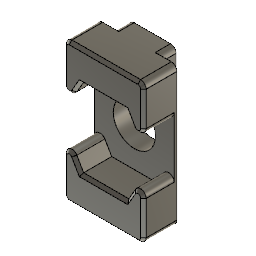
TNut_HeatExpansion v1 (Autodesk Fusion 360 design; units mm, degrees)
Autodesk Fusion 360 part; units mm, degrees
sketch "Sketch1" plane through (0, 0, 0) normal (0, 0, 1) x (1, 0, 0)
  line L0 (-2.85, 0.9) -> (-2.85, -1.5)
  line L1 (2.85, -1.5) -> (2.85, 0.9)
  line L2 (2.85, 0.9) -> (1.7, 0.9)
  line L3 (1.7, 0.9) -> (1.7, 2)
  line L4 (1.7, 2) -> (-1.7, 2)
  line L5 (-1.7, 2) -> (-1.7, 0.9)
  line L6 (-1.7, 0.9) -> (-2.85, 0.9)
  line L7 (-2.85, -1.5) -> (2.85, -1.5)
  dimension "d1" = 3.4
  dimension "d2" = 5.7
  dimension "d3" = 2.4
  dimension "d4" = 1.1
  dimension "d5" = 1.7
  dimension "d6" = 2
  dimension "d7" = 1.15
  constraint vertical L0
  constraint parallel L0 L1
  constraint perpendicular L0 L2
  constraint perpendicular L2 L3
  constraint perpendicular L3 L4
  constraint perpendicular L4 L5
  constraint perpendicular L0 L6
  constraint collinear L2 L6
  constraint perpendicular L0 L7
  measures "d1" distance of L3 L5
  measures "d2" distance of L0 L1
  measures "d3" distance of L0.start L0.end
  measures "d4" distance of L4 L6
  measures "d5" distance of origin L5
  measures "d6" distance of origin L4
  measures "d7" distance of L0 L5
extrude "Extrude1" add sketch "Sketch1" along normal blind 10
sketch "Sketch2" plane through (0, -1.5, 0) normal (0, -1, 0) x (1, 0, 0)
  line L0 (-2.85, 0) -> (2.85, 0)
  line L1 (2.85, 0) -> (2.85, 10)
  line L2 (2.85, 10) -> (-2.85, 10)
  line L3 (-2.85, 10) -> (-2.85, 0)
  line L4 (1.6166, 2.2) -> (3.2332, 5)
  line L5 (3.2332, 5) -> (1.6166, 7.8)
  line L6 (1.6166, 7.8) -> (-1.6166, 7.8)
  line L7 (-1.6166, 7.8) -> (-3.2332, 5)
  line L8 (-3.2332, 5) -> (-1.6166, 2.2)
  line L9 (-1.6166, 2.2) -> (1.6166, 2.2)
  circle A0 centre (0, 5) radius 1.5
  point P0 (0, 5)
  dimension "d10" = 2.8
  dimension "d11" = 2.85
  dimension "d19" = 5
  dimension "d20" = 3
  constraint parallel L2 L6
  constraint coincident P0 A0.centre
  measures "d10" distance of P0 L9
  measures "d11" distance of L3 P0
  measures "d19" distance of L0 P0
  measures "d20" diameter of A0
extrude "Extrude2" cut sketch "Sketch2" against normal blind 2.2 contours L1 L3 L4 L5 L6 L7 L8 L9 | A0
fillet "Fillet1" radius 0.4 4 edges at (-2.85, -0.4, 4.3363) (2.85, -0.4, 5.6637) (2.85, -0.4, 4.3363) (-2.85, -0.4, 5.6637)
fillet "Fillet2" radius 0.4 8 edges at (-1.7, 1.45, 0) (-2.85, -0.3, 0) (-2.85, -0.3, 10) (-1.7, 1.45, 10) (1.7, 1.45, 0) (2.85, -0.3, 0) (1.7, 1.45, 10) (2.85, -0.3, 10)
chamfer "Chamfer1" distance 0.2 angle 45 20 edges at (0, -1.5, 0) (2.7328, -1.5, 0.1172) (2.85, -1.5, 1.6218) (2.5535, -1.5, 3.2299) (1.8601, -1.5, 2.6218) (-1.8601, -1.5, 2.6218) (-2.5535, -1.5, 3.2299) (-2.85, -1.5, 1.6218) (-2.7328, -1.5, 0.1172) (0, -1.5, 2.2) (-2.85, -1.5, 8.3782) (-2.7328, -1.5, 9.8828) (0, -1.5, 10) (2.7328, -1.5, 9.8828) (2.85, -1.5, 8.3782) (2.5535, -1.5, 6.7701) (1.8601, -1.5, 7.3782) (-1.8601, -1.5, 7.3782) (-2.5535, -1.5, 6.7701) (0, -1.5, 7.8)
extrude "Extrude3" cut sketch "Sketch2" against normal blind 5 contours A0
equation "d5 = ( 3.4 / 2 ) * 1 mm"
equation "d7 = ( ( 5.7 - 3.4 ) / 2 ) * 1 mm"
equation "d10 = ( 5.6 / 2 ) * 1 mm"
equation "d11 = ( 5.7 / 2 ) * 1 mm"
